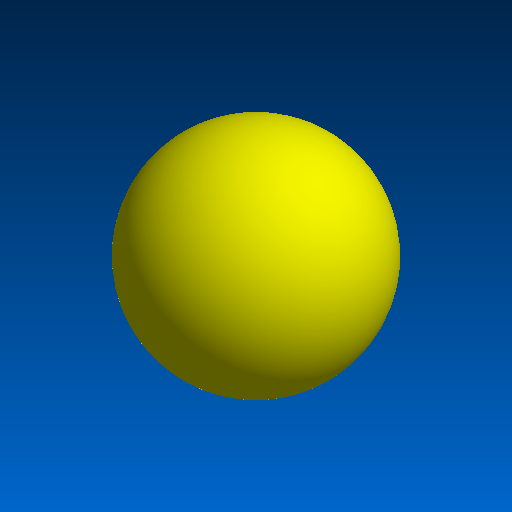
# Autodesk Inventor part: W 606-2Z_PART3
Saved by Autodesk Inventor 2018 (Build 220112000, 112)
## iProperties
Category: PARTsolutions
Company: SKF
Part Number: W 606-2Z_PART3
Material: Stainless Steel
Catalog Web Link: www.cadenas.de
Description: -Deep groove ball bearings
Vendor: SKF
Document SubType Name: Modeling
Designer: partserver
Manufacturer: SKF
Mass: 0.179594 g
Surface Area: 0.384845 cm^2
Volume: 0.0224493 cm^3
Density: 8 g/cm^3
Appearance: Semi-Polished
PSOL_IDENT_0: {$CADENAS_DATA\23d-libs\skf_r32\bearings_units_and_housings\ball_bearings\deep_groove_ball_bearings\
PSOL_IDENT_1: bb1_001_101.prj},195 {VTYP=3D},{NB=W 606-2Z_PART3},{LINA=W 606-2Z_PART3},{NN=BB1_001_101_PART3},{NOP
PSOL_IDENT_2: RJ=TRUE},{DATE=10.06.2020 10:28:41},{GEOMDATE=07.04.2020 07:08:50},{VERSION=},{LINEID=16750},{WBVAR=
PSOL_IDENT_3: },{WBNUMERIC=}  {NB=W 606-2Z_PART3},{LINA=W 606-2Z_PART3},{KT=DUMMY},{DESIGNATION=W 606-2Z},{DD=6.00
PSOL_IDENT_4: 0},{D=17.000},{B=6.000},{C=0.000},{DD1=0.00},{DD2=8.20},{D1=0.00},{D2=14.80},{D3=0.000},{D4=0.000},{
PSOL_IDENT_5: HH=MIN},{BB=0.000},{FF=0.00},{R0MAX=MIN},{R0=MIN},{R12=0.30},{PITCH=11.30},{DW=3.500},{DDAMIN=7.700}
PSOL_IDENT_6: ,{DDAMAX=8.100},{DDBMIN=MIN},{DDBMAX=MIN},{DBMIN=MIN},{DAMAX=15.000},{BBAMIN=MIN},{CAMAX=MIN},{RAMAX=
PSOL_IDENT_7: 0.300},{LOAD1=1.950},{LOAD2=0.830},{LOAD3=0.036},{SPEED1=95000},{SPEED2=48000},{KR=0.030},{F0=11.400
PSOL_IDENT_8: },{Z=6},{II=1},{MASS=0.006},{BEARING=W 606-2Z},{RING=},{HELP=1.677},{HELP2=1.100},{DD1ALG=3.900},{YA
PSOL_IDENT_9: LG=4.513},{PITCH1=11.300},{DW1=3.500},{YALG1=6.823},{HALG1=1.677},{SH=4.100},{CU=0.500},{DESIGN=dgbb
PSOL_IDENT_10: w2z},{HALG=1.5125},{B1=0},{SHIELDHELP=2}
NB: W 606-2Z_PART3
NT: Deep groove ball bearings
NBSYN: $DESIGNATION._PART3
LINA: W 606-2Z_PART3
CATALOG: SKF
SUPPLIER: SKF
ARTICLENO: W 606-2Z_PART3
BOMINFO: W 606-2Z_PART3
CREATOR: CADENAS GmbH
Title: W 606-2Z_PART3
Author: Cadenas PARTsolutions
Comments: Deep groove ball bearings
Autodesk Inventor part; units mm, degrees
ref_plane "YZ Plane" through (0, 0, 0) normal (1, 0, 0) x (0, 1, 0)
ref_plane "XZ Plane" through (0, 0, 0) normal (0, 1, 0) x (-1, 0, 0)
ref_plane "XY Plane" through (0, 0, 0) normal (0, 0, 1) x (1, 0, 0)
sketch "Sketch_6" plane through (0, 0, 0) normal (0, 0, 1) x (1, 0, 0)
  line L0 (4.75, 5.65) -> (1.25, 5.65)
  arc A0 (4.75, 5.65) -> (1.25, 5.65) centre (3, 5.65) ccw
  line L1 (4.75, 5.65) -> (1.25, 5.65)
  dimension "d0" = 360
  constraints: 4 end point, 2 point on circle, 1 centre point
revolve "Revolution1" add sketch "Sketch_6" angle 360 about axis through (4.75, 5.65, 0) along (1, 0, 0)
body "Solid1"
